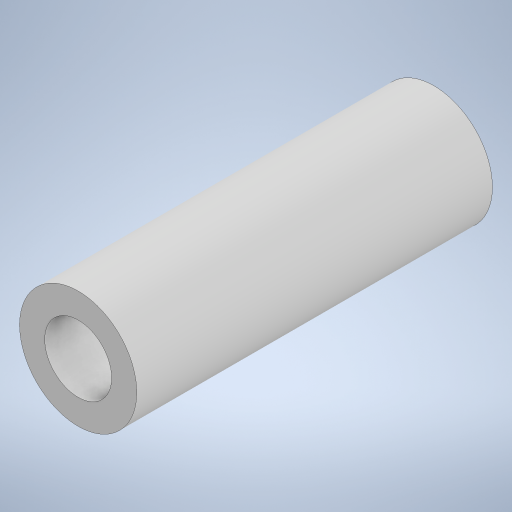
# Autodesk Inventor part: ShaftToScrewCoupler
Saved by Autodesk Inventor 2023 (Build 270158000, 158)
## iProperties
Created: 2023-06-03
Part Number: ShaftToScrewCoupler
Material: Ogólny
Document SubType Name: Modeling
Designer: Kamil
Density: 1 g/cm^3
Appearance: Domyślna
Author: Kamil
Autodesk Inventor part; units mm, degrees
ref_plane "YZ Plane" through (0, 0, 0) normal (1, 0, 0) x (0, 1, 0)
ref_plane "XZ Plane" through (0, 0, 0) normal (0, 1, 0) x (-1, 0, 0)
ref_plane "XY Plane" through (0, 0, 0) normal (0, 0, 1) x (1, 0, 0)
sketch "Szkic1" plane through (0, 0, 0) normal (0, 0, 1) x (1, 0, 0)
  circle A0 centre (0.8001, -1.3838) radius 2.7994
  circle A1 centre (0.8001, -1.3834) radius 1.599
  line L0 (0, -2.7688) -> (0, 0)
  line L1 (0, 0.313) -> (0, -3.3164)
  point P0 (0.8, -1.3844)
  point P1 (0, 0.0011)
  point P2 (0, -2.7679)
  constraints: 4 end point, 2 centre point, 1 vertical
extrude "Wyciągnięcie proste1" add sketch "Szkic1" along normal blind 17
extrude "Wyciągnięcie proste2" add sketch "Szkic1" along normal blind 9 contours L0 A1 picked at (-0.3334, -1.4921)
